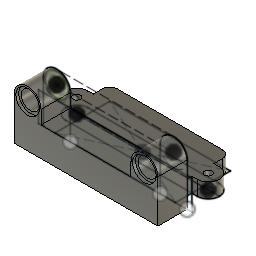
frontsensormount (Autodesk Fusion 360 design; units mm, degrees)
Autodesk Fusion 360 part; units mm, degrees
sketch "Sketch1" plane through (0, 0, 0) normal (0, 0, 1) x (1, 0, 0) in component "Component"
  line L0 (16.5, -7.5) -> (-16.5, -7.5)
  line L1 (-16.5, -7.5) -> (-16.5, 7.5)
  line L2 (-16.5, 7.5) -> (16.5, 7.5)
  line L3 (16.5, 7.5) -> (16.5, -7.5)
  line L4 (16.5, -7.5) -> (-16.5, 7.5) construction
  line L5 (-16.5, -7.5) -> (16.5, 7.5) construction
  line L6 (-18, 0) -> (18, 0) construction
  circle A0 centre (-18, 0) radius 1
  circle A1 centre (-18, 0) radius 1.5 construction
  circle A2 centre (18, 0) radius 1
  circle A3 centre (18, 0) radius 1.5 construction
  line L7 (-18, -3) -> (18, -3)
  arc A4 (18, -3) -> (17.9937, 3) centre (18, 0) ccw
  line L8 (17.9937, 3) -> (-18, 3)
  arc A5 (-18, 3) -> (-18, -3) centre (-18, 0) ccw
  line L9 (-18, 0) -> (18, 0) construction
  line L10 (21, 0.0031) -> (-21, 0)
  dimension "d1" = 33
  dimension "d2" = 15
  dimension "d3" = 36
  dimension "d4" = 2
  dimension "d6" = 7.5
  dimension "d7" = 2
  dimension "d31" = 42
  constraint horizontal L0
  constraint perpendicular L0 L1
  constraint parallel L0 L2
  constraint parallel L1 L3
  constraint coincident L4 origin
  constraint coincident L5 origin
  constraint parallel L2 L6
  constraint coincident L6.start A0.centre
  constraint concentric A0 A1
  constraint coincident L6.end A2.centre
  constraint concentric A2 A3
  constraint tangent L7 A4
  constraint parallel L7 L8
  constraint tangent L7 A5
  constraint parallel L6 L9
  constraint tangent L3 A3
  constraint tangent L1 A1
  constraint equal A1 A3
  constraint tangent L8 A5
  constraint perpendicular L3 L8
  constraint midpoint A4 L10.start
  constraint midpoint A5 L10.end
  measures "d1" distance of L1.end L2.end
  measures "d2" distance of L0.end L1.end
  measures "d3" distance of L6.start L6.end
  measures "d4" diameter of A0
  measures "d6" distance of L2 L6
  measures "d7" diameter of A2
  measures "d31" horizontal distance of L10.start L10.end
extrude "Extrude1" add sketch "Sketch1" along normal blind 4 contours L0 L1 L3 L7 | L1 L3 L7 L10 | L3 A2 L7 A4 L10 | L1 A0 L7 A5 L10 | L1 L3 L8 L10 | L3 A2 A4 L8 L10 | L1 A0 L8 A5 L10 | L1 L2 L3 L8 in component "Component"
sketch "Sketch4" plane through (0, -7.5, 0) normal (0, -1, 0) x (1, 0, 0) in component "Component"
  line L0 (-16.5, 0) -> (16.5, 0)
  line L1 (16.5, 0) -> (16.5, 4)
  line L2 (16.5, 4) -> (-16.5, 4)
  line L3 (-16.5, 4) -> (-16.5, 0)
  circle A0 centre (-16, 11.69) radius 2.52
  circle A1 centre (-16, 11.69) radius 3.22
  line L4 (-16, 8) -> (16, 8)
  arc A2 (16, 8) -> (16, 15.38) centre (16, 11.69) ccw construction
  line L5 (16, 15.38) -> (-16, 15.38) construction
  arc A3 (-16, 15.38) -> (-16, 8) centre (-16, 11.69) ccw construction
  line L6 (-16, 11.69) -> (16, 11.69) construction
  line L7 (-21, 0) -> (21, 0)
  line L8 (21, 0) -> (21, 8)
  line L9 (21, 8) -> (-21, 8)
  line L10 (-21, 8) -> (-21, 0)
  line L11 (-19.69, 11.69) -> (-19.69, 0)
  line L12 (19.69, 11.69) -> (19.69, 0)
  circle A4 centre (-16, 11.69) radius 3.69 construction
  line L13 (-12.31, 11.69) -> (-12.31, -0.0046)
  circle A5 centre (16, 11.69) radius 3.69 construction
  line L14 (12.31, 11.69) -> (12.31, -0.001)
  arc A6 (19.69, 11.69) -> (12.31, 11.69) centre (16, 11.69) ccw
  arc A7 (-12.31, 11.69) -> (-19.69, 11.69) centre (-16, 11.69) ccw
  dimension "d23" = 5.04
  dimension "d24" = 6.44
  dimension "d27" = 7.38
  dimension "d29" = 42
  dimension "d30" = 8
  dimension "d32" = 32
  dimension "d33" = 7.38
  dimension "d34" = 7.38
  constraint tangent L4 A2
  constraint tangent A2 L5
  constraint parallel L4 L5
  constraint tangent L4 A3
  constraint coincident A0.centre A1.centre
  constraint tangent L5 A3
  constraint coincident A2.centre L6.end
  constraint horizontal L7
  constraint vertical L8
  constraint horizontal L9
  constraint vertical L10
  constraint midpoint L0 L7
  constraint midpoint L4 L9
  constraint tangent A2 L9
  constraint parallel L4 L6
  constraint midpoint A3 L11.start
  constraint coincident L7 L11.end
  constraint tangent A3 L11
  constraint perpendicular L7 L11
  constraint midpoint A2 L12.start
  constraint tangent A2 L12
  constraint perpendicular L7 L12
  constraint concentric A3 A4
  constraint vertical L13
  constraint coincident A4 L13.start
  constraint coincident L6 L13.start
  constraint concentric A2 A5
  constraint vertical L14
  constraint coincident L6 L14.start
  constraint coincident A5 L14.start
  constraint tangent L12 A6
  constraint tangent L11 A7
  measures "d23" diameter of A0
  measures "d24" diameter of A1
  measures "d27" distance of L4 L5
  measures "d29" distance of L7.start L7.end
  measures "d30" distance of L7.end L8.end
  measures "d32" distance of A0.centre A2.centre
  measures "d33" diameter of A4
  measures "d34" diameter of A5
extrude "Extrude2" add sketch "Sketch4" along normal blind 8 contours L0 L1 L2 L7 L14 | L0 L2 L7 L13 L14 | L1 L2 L4 L7 L9 L12 L14 | L0 L2 L3 L7 L13 | L2 L4 L9 L13 L14 | L7 L8 L9 L12 | L2 L3 L4 L7 L9 L11 L13 | L4 L9 L12 L14 A6 | L7 L9 L10 L11 | L4 L9 L11 L13 A7 | A0 | A1 in component "Component"
extrude "Extrude3" cut sketch "Sketch4" along normal blind 8 contours A0 in component "Component"
extrude "Extrude4" cut sketch "Sketch4" along normal blind 0.8 contours A1 in component "Component"
ref_plane "WorkPlane1" through (-16, -11.5, 11.69) normal (0, -1, 0) x (1, 0, 0) in component "Component"
mirror "Mirror1" about plane through (-16, -11.5, 11.69) normal (0, -1, 0) of "Extrude4" in component "Component"
ref_plane "WorkPlane2" through (0, -11.5, 4) normal (1, 0, 0) x (0, 0, 1) in component "Component"
mirror "Mirror2" about plane through (0, -11.5, 4) normal (1, 0, 0) of "Extrude3", "Extrude4", "Mirror1" in component "Component"
extrude "Extrude5" cut 2 faces at (20.1267, -12.8333, 8) (-20.1267, -10.1667, 8) along direction (0, 0, -1) blind 8 in component "Component"
fillet "Fillet1" radius 2 2 edges at (-16.5, 7.5, 2) (16.5, 7.5, 2) in component "Component"
component "Component" placed x (1, 0, 0) y (0, 1, 0) z (0, 0, 1) at (0, 0, 0)
equation "d23 = 4.8 mm + 0.24 mm"
equation "d24 = 6.2 mm + 0.24 mm"
